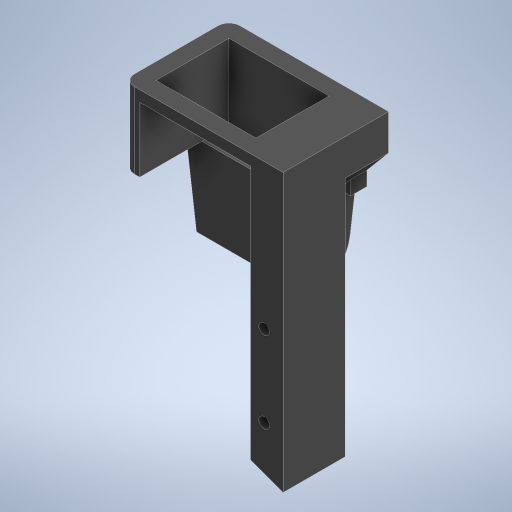
# Autodesk Inventor part: switch_setter
Saved by Autodesk Inventor 2024.1 (Build 281209000, 209)
## iProperties
Created: 2024-02-15
Part Number: switch_setter
Material: 一般
Document SubType Name: Modeling
Designer: hibik
Density: 1 g/cm^3
Appearance: 既定
Author: hibik
Autodesk Inventor part; units mm, degrees
note: some values were not read from the file. Chosen so that the rebuilt part matches the saved one: edges of "フィレット3".
ref_plane "YZ Plane" through (0, 0, 0) normal (1, 0, 0) x (0, 1, 0)
sketch "スケッチ1" plane through (0, 0, 0) normal (1, 0, 0) x (0, 1, 0)
  line L0 (45, 0) -> (0, 0)
  line L1 (0, 0) -> (0, -11.5)
  line L2 (0, -11.5) -> (45, -11.5)
  line L3 (45, -11.5) -> (45, 0)
  dimension "d0" = 45
  dimension "d1" = 11.5
  constraints: 8 end point, 2 parallel, 1 coincident, 1 horizontal, 1 perpendicular
  measures "d0" distance of L0.start L0.end
  measures "d1" distance of L2.end L0.start
extrude "押し出し1" add sketch "スケッチ1" along normal blind 3
sketch "スケッチ5" plane through (0, 45, 0) normal (0, 1, 0) x (1, 0, 0)
  line L0 (-5, 3) -> (-23.5, 3)
  line L1 (-23.5, 3) -> (-23.5, 16.5)
  line L2 (-23.5, 16.5) -> (-5, 16.5)
  line L3 (-5, 16.5) -> (-5, 3)
  line L4 (0, 0) -> (-26.5, 0)
  line L5 (-26.5, 0) -> (-26.5, 19.5)
  line L6 (-26.5, 19.5) -> (0, 19.5)
  line L7 (0, 19.5) -> (0, 0)
  point P0 (3, 0)
  dimension "d15" = 18.5
  dimension "d16" = 13.5
  dimension "d17" = 3
  dimension "d18" = 5
  dimension "d19" = 3
  dimension "d20" = 3
  constraints: 16 end point, 4 parallel, 2 horizontal, 2 perpendicular, 1 coincident
  measures "d15" distance of L1.end L2.end
  measures "d16" distance of L0.end L1.end
  measures "d17" distance between parallel lines of L4 L0
  measures "d18" distance between parallel lines of L7 L3
  measures "d19" distance between parallel lines of L5 L1
  measures "d20" distance between parallel lines of L6 L2
extrude "押し出し4" add sketch "スケッチ5" against normal blind 2
ref_plane "作業平面1" through (0, 45, -9.5) normal (1, 0, 0) x (0, 0, -1)
sketch "スケッチ7" plane through (0, 45, -9.5) normal (1, 0, 0) x (0, 0, -1)
  line L0 (0, 0) -> (10, 0) projected
  line L1 (10, -2) -> (2, -2) projected
  line L2 (10, 0) -> (10, -2) projected
  line L3 (2, 0) -> (10, 0) projected
  line L4 (2, -2) -> (2, 0) projected
  point P0 (-9.5, -45)
extrude "押し出し6" cut sketch "スケッチ7" against normal blind 1
fillet "フィレット2" radius 2 2 edges at (-26.5, 44, 0) (-26.5, 44, -19.5)
sketch "スケッチ8" plane through (0, 0, 0) normal (-1, 0, 0) x (0, 0, 1)
  line L0 (0, 43) -> (-11.5, 43) projected
  line L1 (-11.5, 0) -> (-11.5, 43) projected
  line L2 (0, 0) -> (-11.5, 0) projected
  line L3 (0, 43) -> (0, 0) projected
  line L4 (-3, 39.3409) -> (0, 39.3409)
  line L5 (0, 39.3409) -> (0, 27.7002)
  line L6 (0, 27.7002) -> (-3, 27.7002)
  line L7 (-3, 27.7002) -> (-3, 39.3409)
  constraints: 8 end point, 2 parallel, 1 horizontal, 1 perpendicular
extrude "押し出し7" add sketch "スケッチ8" along normal blind 3
ref_plane "作業平面2" through (3, 2, -11.5) normal (0, 0, -1) x (-1, 0, 0)
sketch "スケッチ10" plane through (3, 2, -11.5) normal (0, 0, -1) x (-1, 0, 0)
  line L0 (-2, -9) -> (6, -6) projected
  line L1 (6, -6) -> (6, 22) projected
  line L2 (0, -2) -> (0, 0) projected
  line L3 (0, -2) -> (6, -2) projected
  line L4 (0, -2) -> (0, -8.25)
  point P0 (3, -2)
  constraints: 2 end point, 1 point on line, 1 vertical
extrude "押し出し9" add sketch "スケッチ10" against normal up to surface (11.5 mm away)
sketch "スケッチ11" plane through (3, 45, -11.5) normal (0, 0, -1) x (-1, 0, 0)
  circle A0 centre (3.5, -26.8338) radius 1 projected
  circle A1 centre (3.5, -41.8338) radius 1 projected
  point P0 (3, -45)
sketch "スケッチ12" plane through (0, 43, 0) normal (0, -1, 0) x (1, 0, 0)
  line L0 (-1, -11.5) -> (-3, -11.5) projected
  line L1 (-3, -11.5) -> (-3, 0) projected
  line L2 (-3, 0) -> (-24.5, 0) projected
  arc A0 (-24.5, 0) -> (-26.5, -2) centre (-24.5, -2) ccw projected
  line L3 (-26.5, -2) -> (-26.5, -17.5) projected
  arc A1 (-26.5, -17.5) -> (-24.5, -19.5) centre (-24.5, -17.5) ccw projected
  line L4 (-24.5, -19.5) -> (-1, -19.5) projected
  line L5 (-1, -19.5) -> (-1, -11.5) projected
  line L6 (-23.5, -3) -> (-5, -3) projected
  line L7 (-5, -3) -> (-5, -16.5) projected
  line L8 (-5, -16.5) -> (-23.5, -16.5) projected
  line L9 (-23.5, -16.5) -> (-23.5, -3) projected
  line L10 (-5, -16.5) -> (-1, -16.5)
  line L11 (-23.5, -3) -> (-23.5, 0)
  line L12 (-3, -11.5) -> (-5, -16.5)
  point P0 (0, 0)
  constraints: 6 end point, 2 point on line, 1 horizontal, 1 perpendicular
extrude "押し出し10" add sketch "スケッチ12" along normal blind 12 contours L5 L4 A1 L3 A0 L2 L11 L9 L8 L10
sketch "スケッチ13" plane through (3, 45, -11.5) normal (0, 0, -1) x (-1, 0, 0)
  line L0 (6, -16.8338) -> (-2.2366, -7.0996) projected
  line L1 (6, -2) -> (6, -49) projected
  line L2 (4, -2) -> (6, -2) projected
  line L3 (4, -2) -> (4, 0) projected
  line L4 (4, 0) -> (0, 0) projected
  line L5 (0, 0) -> (0, -51.25) projected
  line L6 (0, -51.25) -> (6, -49) projected
  line L7 (0, -6.6466) -> (6, -13.7375)
  line L8 (6, -49) -> (6, -2) projected
  point P0 (3, -45)
  point P1 (6, -13.7375)
  dimension "d38" = 2
  constraints: 2 end point, 2 point on line, 1 parallel
  measures "d38" distance between parallel lines of L7 L0
extrude "押し出し11" add sketch "スケッチ13" along normal up to surface (8 mm away) contours L7 L5 L4 L3 L2 L1
sketch "スケッチ14" plane through (0, 31, 0) normal (0, -1, 0) x (1, 0, 0)
  line L0 (-1, -19.5) -> (-1, -16.5) projected
  line L1 (-1, -16.5) -> (-23.5, -16.5) projected
  line L2 (-23.5, -16.5) -> (-23.5, 0) projected
  line L3 (-23.5, 0) -> (-24.5, 0) projected
  arc A0 (-24.5, 0) -> (-26.5, -2) centre (-24.5, -2) ccw projected
  line L4 (-26.5, -2) -> (-26.5, -17.5) projected
  arc A1 (-26.5, -17.5) -> (-24.5, -19.5) centre (-24.5, -17.5) ccw projected
  line L5 (-24.5, -19.5) -> (-1, -19.5) projected
  line L6 (-1, -19.5) -> (-26.5, -19.5)
  line L7 (-26.5, -19.5) -> (-26.5, -11.5)
  line L8 (-26.5, -11.5) -> (-1, -11.5)
  line L9 (-1, -11.5) -> (-1, -19.5)
  line L10 (-3, -11.5) -> (-3, -16.5) projected
  line L11 (-3, -16.5) -> (-3, -19.5)
  point P0 (0, 0)
  dimension "d41" = 8
  constraints: 10 end point, 2 parallel, 2 perpendicular, 2 point on line, 1 horizontal
  measures "d41" distance between parallel lines of L5 L8
extrude "押し出し12" add sketch "スケッチ14" along normal blind 15 contours L5 A1 L4 L8 L2 L1 L11 | L1 L2 L8 L10
chamfer "面取り1" distance 2 distance2 15 3 edges at (-13.75, 16, -19.5) (-25.9142, 16, -18.9142) (-26.5, 16, -14.5) measured on face at (-18, 16, -14.1667)
fillet "フィレット3" radius 8 1 edges at (-13.75, 16, -17.5001)
extrude "押し出し13" cut sketch "スケッチ11" against normal through all
equation "\"d19\" = d17"
equation "\"d20\" = d17"
